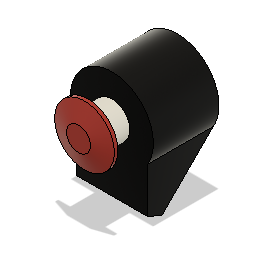
Emergency Button Case v5 (Autodesk Fusion 360 design; units mm, degrees)
Autodesk Fusion 360 part; units mm, degrees
box "BoxPrimitive1" add length 35 width 60 height 55 placed x (0, 1, 0) y (-1, 0, 0) z (0, 0, 1) at (60, 0, 0) makes body 1
sketch "Sketch2" plane through (0, 0, 55) normal (0, 0, 1) x (1, 0, 0)
  line L0 (60, 35) -> (0, 35)
  line L1 (0, 35) -> (0, 0)
  line L2 (0, 0) -> (60, 0)
  line L3 (60, 0) -> (60, 35)
  circle A0 centre (30, 17.5) radius 34.7311
  constraint coincident L1.end A0
  constraint coincident L0.start A0
  constraint coincident L2.end A0
extrude "Extrude1" add sketch "Sketch2" against normal blind 55 contours L3 A0 | L0 A0 | L1 A0 bodies 1
shell "Shell1" thickness 3 removed faces 1 at (26.5805, 16.8939, 0) on bodies 1
sketch "Sketch3" plane through (0, 0, 55) normal (0, 0, 1) x (1, 0, 0)
  line L0 (0, 0) -> (60, 0)
  arc A0 (60, 0) -> (0, 0) centre (30, 17.5) ccw
  line L1 (0, 0) -> (60, 0)
  line L2 (60, 0) -> (60, 35)
  line L3 (60, 35) -> (0, 35)
  line L4 (0, 35) -> (0, 0)
  circle A1 centre (30, 17.5) radius 11.5
  dimension "d10" = 23
  constraint horizontal L1
  constraint vertical L2
  constraint horizontal L3
  constraint vertical L4
  constraint coincident A0 L2.end
  constraint coincident L0.start A0.end
  constraint coincident L0.end A0.start
  constraint concentric A0 A1
  measures "d10" diameter of A1
extrude "Extrude2" cut sketch "Sketch3" against normal blind 3 contours A1 bodies 1
extrude "Extrude10" add 1 faces at (40, 0, 18.3333) along direction (0, -1, 0) blind 55 on bodies 1 bodies 1
sketch "Sketch12" plane through (0, 0, 0) normal (-1, 0, 0) x (0, 0, 1)
  line L0 (55, 0) -> (0, 0)
  line L1 (0, 0) -> (0, -55)
  line L2 (0, -55) -> (55, -55)
  line L3 (55, -55) -> (55, 0)
  line L4 (0, 0) -> (55, -55)
  line L5 (0, 0) -> (77.7817, 0) construction
  dimension "d62" = 45
  constraint horizontal L5
  constraint coincident L0.end L1.start
  constraint coincident L2 L3.start
  measures "d62" angle of L4 L5
extrude "Extrude11" cut sketch "Sketch12" against normal blind 60 contours L1 L2 L4 bodies 1
sketch "Sketch15" plane through (0, 0, 0) normal (0, -0.707107, -0.707107) x (-1, 0, 0)
  line L0 (0, -77.7817) -> (0, 0)
  line L1 (0, 0) -> (-60, 0)
  line L2 (-60, 0) -> (-60, -77.7817)
  line L3 (-60, -77.7817) -> (0, -77.7817)
  circle A0 centre (-48, -19.7817) radius 1.25
  circle A1 centre (-36, -19.7817) radius 1.25
  circle A2 centre (-24, -19.7817) radius 1.25
  circle A3 centre (-12, -19.7817) radius 1.25
  circle A4 centre (-48, -52.7817) radius 1.25
  circle A5 centre (-36, -52.7817) radius 1.25
  circle A6 centre (-24, -52.7817) radius 1.25
  circle A7 centre (-12, -52.7817) radius 1.25
  dimension "d85" = 12
  dimension "d86" = -33
  dimension "d87" = 12
  dimension "d88" = 12
  dimension "d89" = 25
  dimension "d90" = 2.5
  measures "d87" distance of L2 A0.centre
  measures "d88" distance of L0 A3.centre
  measures "d89" distance of L3 A4.centre
  measures "d90" diameter of A0
extrude "Extrude14" cut sketch "Sketch15" against normal blind 10 contours A0 | A1 | A2 | A3 | A4 | A5 | A6 | A7 bodies 1
chamfer "Chamfer7" distance 17 angle 45 1 edges at (30, -55, 55) on bodies 1
cylinder "CylinderPrimitive1" add diameter 30 height 20 placed x (1, 0, 0) y (0, 1, 0) z (0, 0, 1) at (30, 17.5, 55) separate body makes body 2
cylinder "CylinderPrimitive2" add diameter 50 height 8 placed x (1, 0, 0) y (0, 1, 0) z (0, 0, 1) at (30, 17.5, 75) bodies 2
chamfer "Chamfer8" distance 15 distance2 5 1 edges at (6.6918, 8.4596, 83) measured on face at (23.2241, 16.258, 83) on bodies 2
